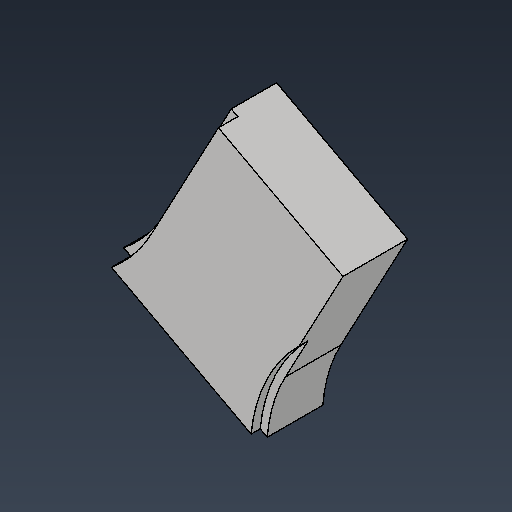
# Autodesk Inventor part: bearing_cap
Saved by Autodesk Inventor 2026.2 (Build 302298010, 298A)
## iProperties
Created: 2026-04-04
Part Number: bearing_cap
Material: Generic
Document SubType Name: Modeling
Designer: szymo
Density: 1 g/cm^3
Appearance: Default
Author: szymo
Autodesk Inventor part; units mm, degrees
ref_plane "YZ Plane" through (0, 0, 0) normal (1, 0, 0) x (0, 1, 0)
ref_plane "XZ Plane" through (0, 0, 0) normal (0, 1, 0) x (-1, 0, 0)
ref_plane "XY Plane" through (0, 0, 0) normal (0, 0, 1) x (1, 0, 0)
ref_plane "Work Plane1" through (2.4666, 0.1565, -5.1) normal (0, 0, 1) x (0.4710614, 0.8821004, 0)
sketch "Sketch1" plane through (2.4666, 0.1565, -5.1) normal (0, 0, 1) x (0.4710614, 0.8821004, 0)
  line L0 (11.7, -17.8967) -> (11.7, 22.3967)
  line L1 (-8.3, -5.688) -> (-8.3, 9.6856)
  line L2 (-2.8, -4.5491) -> (9.7, -4.5491)
  line L3 (9.7, -4.5491) -> (9.7, 8.5467)
  line L4 (9.7, 8.5467) -> (-2.8, 8.5467)
  circle A0 centre (-2.8, -18.3991) radius 13.85 projected
  circle A1 centre (-2.8, -18.3991) radius 14.5 projected
  circle A2 centre (-2.8, 22.3967) radius 14.5 projected
  circle A3 centre (-2.8, 22.3967) radius 13.85 projected
  circle A4 centre (-1.3, 2.1021) radius 5 projected
  line L5 (-2.8, 7.8967) -> (9.7, 7.8967)
  point P0 (-1.3, 2.1021)
  dimension "d1" = 2
  dimension "d19" = 2
  constraints: 12 end point, 5 point on circle, 4 perpendicular, 4 tangent, 2 vertical, 1 point on line
  measures "d1" distance between parallel lines of L3 L0
  measures "d19" distance edge to line of A4 L1
ref_plane "Work Plane2" through (-46.3211, -19.4757, -1.1) normal (0, 0, -1) x (-0.2419299, 0.9702937, 0)
extrude "Extrusion1" add sketch "Sketch1" along normal up to surface (4 mm away) contours L1 A1 L2 A0 | L1 A2 L5 L3 L2 A1 | L1 A3 L4 A2 | A2 L4 L3 L5 picked at (-1.0277, -4.3445) picked at (-0.4071, 8.4267)
ref_plane "Work Plane4" through (-8.352, -36.71, -0.2) normal (0, 0, -1) x (0.0887638, 0.9960527, 0)
sketch "Sketch6" plane through (-9.9869, -2.6024, -1.1) normal (0, 0, 1) x (0.8821004, -0.4710614, 0)
  circle A0 centre (7.5835, 7) radius 5 projected
  line L0 (14.2347, 18) -> (1.1389, 18) projected
  line L1 (1.1389, 18) -> (1.1389, 5.5) projected
  arc A1 (0, 0) -> (1.1389, 5.5) centre (-12.7111, 5.5) ccw projected
  line L2 (0, 0) -> (15.3736, 0) projected
  arc A2 (14.2347, 5.5) -> (15.3736, 0) centre (28.0847, 5.5) ccw projected
  line L3 (14.2347, 5.5) -> (14.2347, 18) projected
  circle A3 centre (-12.7111, 5.5) radius 14.5 projected
  line L4 (1.7889, 5.5) -> (1.7889, 18)
  point P0 (7.5835, 7)
  point P1 (0.7053, 0)
  constraints: 2 end point, 1 perpendicular, 1 point on line, 1 vertical, 2 other
extrude "Extrusion5" add sketch "Sketch6" along normal up to surface (0.9 mm away) contours L3 A2 L2 A3 L4 L0
sketch "Sketch8" plane through (-9.3647, -2.9346, -0.2) normal (0, 0, 1) x (0.8821004, -0.4710614, 0)
  circle A0 centre (6.8782, 7) radius 5 projected
  line L0 (13.5294, 5.5) -> (13.5294, 18) projected
  line L1 (13.5294, 18) -> (1.0836, 18) projected
  line L2 (1.0836, 18) -> (1.0836, 5.5) projected
  arc A1 (0, 0) -> (1.0836, 5.5) centre (-13.4164, 5.5) ccw projected
  line L3 (0, 0) -> (14.6683, 0) projected
  arc A2 (13.5294, 5.5) -> (14.6683, 0) centre (27.3794, 5.5) ccw projected
  circle A3 centre (27.3794, 5.5) radius 14.5 projected
  arc A4 (0, 0) -> (1.0836, 5.5) centre (-13.4164, 5.5) ccw projected
  point P0 (6.8782, 7)
  point P1 (13.963, 0)
  point P2 (13.5294, 9.7927)
extrude "Extrusion6" add sketch "Sketch8" along normal blind 0.4 contours A3 L3 A1 L2 L1 L0
sketch "Sketch9" plane through (-9.3647, -2.9346, 0.2) normal (0, 0, 1) x (0.8821004, -0.4710614, 0)
  arc A0 (0, 0) -> (1.0836, 5.5) centre (-13.4164, 5.5) ccw projected
  line L0 (0, 0) -> (13.963, 0) projected
  arc A1 (13.5294, 9.7927) -> (13.963, 0) centre (27.3794, 5.5) ccw projected
  line L1 (13.5294, 9.7927) -> (13.5294, 18) projected
  line L2 (13.5294, 18) -> (1.0836, 18) projected
  line L3 (1.0836, 18) -> (1.0836, 5.5) projected
  circle A2 centre (6.8782, 7) radius 5 projected
  point P0 (6.8782, 7)
extrude "Extrusion7" add sketch "Sketch9" along normal blind 0.4 contours A0 L3 L2 L1 A1 L0 | A2
body "Solid1"
